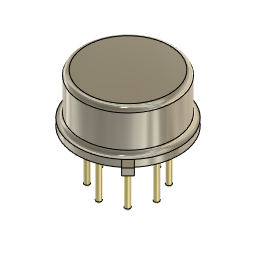
TO-99 (Autodesk Fusion 360 design; units mm, degrees)
Autodesk Fusion 360 part; units mm, degrees
ref_plane "WorkPlane1" through (0, 0, 1) normal (0, 0, 1) x (1, 0, 0)
sketch "Sketch1" plane through (0, 0, 1) normal (0, 0, 1) x (1, 0, 0)
  circle A0 centre (0, 0) radius 2.54 construction
  circle A1 centre (-2.5399, 0.0224) radius 0.225
  circle A2 centre (-1.8118, -1.7802) radius 0.225
  circle A3 centre (-0.0224, -2.5399) radius 0.225
  circle A4 centre (1.7802, -1.8118) radius 0.225
  circle A5 centre (2.5399, -0.0224) radius 0.225
  circle A6 centre (1.8118, 1.7802) radius 0.225
  circle A7 centre (0.0224, 2.5399) radius 0.225
  circle A8 centre (-1.7802, 1.8118) radius 0.225
  dimension "d1" = 5.08
  dimension "d2" = 0.45
  dimension "d4" = 360
  constraint coincident A0.centre origin
  constraint coincident A0 A1.centre
  measures "d1" diameter of A0
  measures "d2" diameter of A1
extrude "Extrude1" add sketch "Sketch1" along normal blind -4.6 and the other way blind -0.2 makes body 1 at (2.0357, 1.7578, -0.4) makes body 2 at (-1.5879, -1.8026, -0.4) makes body 3 at (-2.316, 0, -0.4) makes body 4 at (2.7638, -0.0448, -0.4) makes body 5 at (0.2463, 2.5175, -0.4) makes body 6 at (0.2015, -2.5623, -0.4) makes body 7 at (-1.5563, 1.7894, -0.4) makes body 8 at (2.004, -1.8342, -0.4)
fillet "Fillet4" radius 0.225 8 faces at (1.9893, 1.7476, -3.6) (-1.6359, -1.799, -3.6) (-2.6141, 0.0336, -3.6) (2.4657, -0.0112, -3.6) (0.009, 2.4813, -3.6) (-0.0584, -2.6018, -3.6) (-1.7719, 1.9438, -3.6) (1.8032, -1.9005, -3.6) on bodies 1 2 3 4 5 6 7 8
sketch "Sketch2" plane through (0, 0, 1) normal (0, 0, 1) x (1, 0, 0)
  circle A0 centre (0, 0) radius 4.4775
  circle A1 centre (0, 0) radius 4.065
  line L0 (0, 0) -> (5.001, -5.001) construction
  line L1 (0, 0) -> (7.0725, 0) construction
  line L2 (-0.9476, 0.3925) -> (7.0725, 0.3925) construction
  line L3 (3.4314, -2.8763) -> (4.0906, -3.5355)
  line L4 (0.9476, -0.3925) -> (7.0725, -0.3925) construction
  line L5 (3.5355, -4.0906) -> (4.0906, -3.5355)
  line L6 (2.8763, -3.4314) -> (3.5355, -4.0906)
  circle A2 centre (0, 0) radius 1.905
  circle A3 centre (0, 0) radius 3.5
  dimension "d8" = 8.955
  dimension "d9" = 8.13
  dimension "d18" = 45
  dimension "d21" = 0.915
  dimension "d24" = 3.81
  constraint coincident A0.centre A1.centre
  constraint concentric A0 A1
  constraint horizontal L1
  constraint perpendicular L3 L5
  constraint parallel L0 L3
  constraint parallel L1 L4
  constraint coincident A0 L3.start
  constraint parallel L1 L2
  constraint coincident A0 L6.start
  measures "d8" diameter of A0
  measures "d9" diameter of A1
  measures "d18" angle of L0 L1
  measures "d21" distance of A0 L5
  measures "d24" diameter of A2
extrude "Extrude2" add sketch "Sketch2" along normal blind 0.6 separate body contours A0 makes body 9
extrude "Extrude3" add sketch "Sketch2" along normal blind 4.255 contours A1 | A2 | A3 bodies 9
fillet "Fillet1" radius 0.413 1 edges at (-3.7899, 1.47, 1.6) on bodies 9
fillet "Fillet2" radius 0.413 1 edges at (-3.7899, -1.47, 5.255) on bodies 9
extrude "Extrude4" add sketch "Sketch2" along normal blind 0.6 contours A0 L3 L5 L6 bodies 9
extrude "Extrude5" add sketch "Sketch2" along normal blind -1 and the other way blind -0.2 separate body contours A2 makes body 10
extrude "Extrude6" cut sketch "Sketch2" along normal blind 0.2 contours A2 | A3 bodies 9
fillet "Fillet3" radius 0.2 1 edges at (-3.2631, -1.2657, 1) on bodies 9
chamfer "Chamfer1" distance 0.3 angle 45 1 edges at (-1.7761, 0.6889, 0) on bodies 10
equation "d1 = ( 2.54 * 2 ) * 1 mm"
equation "d6 = -1 mm - 1.6 mm - 2 mm"
equation "d24 = ( ( 4.06 + 3.56 ) / 2 ) * 1 mm"
